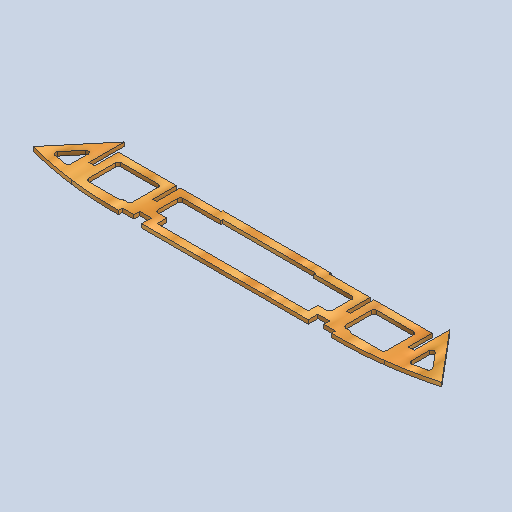
# Autodesk Inventor part: bulkhead_b2
Saved by Autodesk Inventor 2022 (Build 260153070, 153G)
## iProperties
Created: 2021-04-24
Part Number: bulkhead_b2
Material: Plywood, Sheathing, Glazed
Document SubType Name: Modeling
Designer: kardo
Density: 0.75 g/cm^3
Appearance: Plywood - New(2)
Mass: 3.53405 g
Surface Area: 67.3675 cm^2
Volume: 4.71206 cm^3
Author: kardo
Autodesk Inventor part; units mm, degrees
ref_plane "YZ Plane" through (0, 0, 0) normal (1, 0, 0) x (0, 1, 0)
ref_plane "XZ Plane" through (0, 0, 0) normal (0, 1, 0) x (-1, 0, 0)
ref_plane "XY Plane" through (0, 0, 0) normal (0, 0, 1) x (1, 0, 0)
derived "frame_outline.ipt"
sketch "bh_b2" plane through (0, -242, 0) normal (0, 1, 0) x (-1, 0, 0)
  line L0 (0, 19.8309) -> (-30, 19.8309) construction
  line L1 (-30, 19.8309) -> (-30, 20.6564) construction
  line L2 (-30, 20.6564) -> (-81, 20.6564) construction
  line L3 (-81, 20.6564) -> (-81, 10.5173) construction
  line L4 (-81, 10.5173) -> (-106.9114, 41.3973) construction
  line L5 (-105.4998, 40.9597) -> (-81, 11.7619)
  line L6 (0, 20.6309) -> (-28, 20.6309)
  line L7 (-28, 20.6309) -> (-28, 21.4564)
  line L8 (-28, 21.4564) -> (-81, 21.4564)
  line L9 (0, 47.4037) -> (0, 20.6309)
  line L10 (-81, 21.4564) -> (-81, 11.7619)
  spline S0 degree 3 poles (-81, 46.6843) (-83.3296, 46.3773) (-85.8016, 46.0077) (-94.6879, 44.4818) (-100.8447, 43.1089) (-106.9114, 41.3973) knots 2.001746 2.001746 2.001746 2.001746 2.383442 2.383442 3.297577 3.297577 3.297577 3.297577
  spline S1 degree 3 poles (-55, 48.2037) (-56.5728, 48.2037) (-58.0596, 48.1988) (-64.6088, 48.1191) (-71.6624, 47.915) (-81, 46.6843) knots 0 0 0 0 0.47184 0.47184 2.001746 2.001746 2.001746 2.001746
  spline S2 degree 3 poles (0, 48.2037) (-9.1667, 48.2037) (-18.3333, 48.2037) (-36.6667, 48.2037) (-45.8333, 48.2037) (-55, 48.2037) knots 0 0 0 0 2.75 2.75 5.5 5.5 5.5 5.5
  spline S3 degree 3 poles (0, 47.4037) (-1.5278, 47.4037) (-4.5833, 47.4037) (-8.4028, 47.4037) (-12.2222, 47.4037) (-15.2778, 47.4037) (-19.0972, 47.4037) (-22.1528, 47.4037) (-25.9722, 47.4037) (-29.0278, 47.4037) (-32.8472, 47.4037) (-35.9028, 47.4037) (-40.4861, 47.4037) (-46.5972, 47.4037) (-51.9444, 47.4037) (-55, 47.4037) knots 0 0 0 0 0.458333 0.916667 1.145833 1.604167 1.833333 2.291667 2.520833 2.979167 3.208333 3.666667 3.895833 4.583333 5.5 5.5 5.5 5.5
  spline S4 degree 3 poles (-55, 47.4037) (-55.2777, 47.4037) (-55.8277, 47.4034) (-56.5054, 47.402) (-57.1788, 47.3996) (-57.7152, 47.3969) (-58.3187, 47.3928) (-58.722, 47.3894) (-59.1266, 47.3854) (-59.3974, 47.3824) (-59.7371, 47.3783) (-60.0133, 47.3747) (-60.3642, 47.3696) (-60.6495, 47.3651) (-61.0842, 47.3576) (-61.5281, 47.3491) (-62.2112, 47.3344) (-62.8367, 47.3188) (-63.6418, 47.2958) (-64.3045, 47.2744) (-65.3265, 47.2372) (-66.386, 47.1927) (-68.0464, 47.1096) (-69.5986, 47.0164) (-71.6355, 46.871) (-73.3429, 46.7297) (-75.5759, 46.5174) (-77.9084, 46.268) (-79.8817, 46.0248) (-80.8955, 45.8912) knots 0 0 0 0 0.083406 0.166812 0.208515 0.291921 0.333624 0.396179 0.41703 0.458733 0.479585 0.521288 0.542139 0.583842 0.604694 0.667249 0.708952 0.792358 0.834061 0.917467 0.95917 1.084279 1.167685 1.334497 1.417903 1.584715 1.668121 1.834933 2.001746 2.001746 2.001746 2.001746
  spline S5 degree 3 poles (-80.8955, 45.8912) (-81.5213, 45.8087) (-82.7935, 45.6346) (-84.4358, 45.3927) (-85.865, 45.1704) (-86.7205, 45.0322) (-87.4128, 44.9174) (-87.7609, 44.8589) (-88.1986, 44.7845) (-88.5505, 44.7239) (-88.9894, 44.6474) (-89.3405, 44.5854) (-89.8666, 44.4914) (-90.3922, 44.396) (-91.1795, 44.2502) (-91.8784, 44.1178) (-92.9251, 43.9148) (-93.9698, 43.706) (-95.5329, 43.382) (-96.9184, 43.0821) (-98.9907, 42.6143) (-101.7434, 41.9582) (-104.1368, 41.3335) (-105.4998, 40.9597) knots 2.001746 2.001746 2.001746 2.001746 2.104714 2.207682 2.259166 2.323522 2.336393 2.362135 2.375006 2.400748 2.413619 2.439361 2.452232 2.490845 2.516587 2.568071 2.593813 2.67104 2.722524 2.825492 2.876976 3.031429 3.237366 3.237366 3.237366 3.237366
  point P0 (0, 0)
  point P1 (-81, 33.6806)
extrude "Extrusion1" add sketch "bh_b2" along normal blind 2
sketch "Sketch2" plane through (0, -242, 47.4037) normal (0, -1, 0) x (1, 0, 0)
  line L0 (81, -35.6418) -> (81, -25.9472) projected
  line L1 (81, -25.9472) -> (81, -13.7231)
  line L2 (81, -13.7231) -> (84, -13.7231)
  line L3 (84, -13.7231) -> (84, -32.0665)
  line L4 (105.4998, -6.444) -> (81, -35.6418) projected
  point P0 (0, -47.4037)
  dimension "d3" = 3
  constraints: 6 end point, 2 point on line, 1 collinear, 1 horizontal, 1 parallel
  measures "d3" distance between parallel lines of L3 L0
sketch "Sketch3" plane through (0, -242, 47.4037) normal (0, -1, 0) x (1, 0, 0)
  line L0 (0, 0) -> (55, 0) projected
  line L1 (0, 0) -> (55, 0) projected
  line L2 (55, 0) -> (55, -2)
  line L3 (55, -2) -> (49, -2)
  line L4 (49, -2) -> (49, -5)
  line L5 (49, -5) -> (43, -5)
  line L6 (43, -5) -> (43, 0)
  point P0 (0, -47.4037)
  dimension "d4" = 5
  dimension "d5" = 2
  dimension "d6" = 6
  dimension "d7" = 6
  constraints: 10 end point, 3 vertical, 2 horizontal, 1 point on line
  measures "d4" distance of L5.end L6.end
  measures "d5" distance of L0.end L2.end
  measures "d6" distance of L2.end L3.end
  measures "d7" distance of L4.end L5.end
extrude "Extrusion2" cut sketch "Sketch2" against normal through all
extrude "Extrusion3" cut sketch "Sketch3" against normal through all
sketch "Sketch4" plane through (0, -242, 20.6309) normal (0, -1, 0) x (1, 0, 0)
  line L0 (84, 13.0497) -> (84, -5.2937) projected
  line L1 (105.4998, 20.3288) -> (84, -5.2937) projected
  line L2 (88, 20.1303) -> (88, 5.6962)
  line L3 (88, 5.6962) -> (98.344, 18.0237)
  line L4 (98.344, 18.0237) -> (88, 20.1303)
  line L5 (88, 20.1303) -> (88.7982, 24.0498)
  line L6 (98.344, 18.0237) -> (99.1422, 21.9433)
  point P0 (0, -20.6309)
  dimension "d13" = 4
  dimension "d14" = 4
  dimension "d15" = 4
  constraints: 10 end point, 3 parallel, 2 perpendicular, 3 other
  measures "d13" distance of L3.end L6.end
  measures "d14" distance between parallel lines of L1 L3
  measures "d15" distance between parallel lines of L0 L2
sketch "Sketch5" plane through (0, -242, 20.6309) normal (0, -1, 0) x (1, 0, 0)
  line L0 (55, 26.7728) -> (55, 24.7728) projected
  line L1 (81, 0.8256) -> (81, 13.0497) projected
  line L2 (81, 0.8256) -> (28, 0.8256) projected
  line L3 (55, 20.7728) -> (55, 4.8256)
  line L4 (55, 4.8256) -> (77, 4.8256)
  line L5 (77, 4.8256) -> (77, 21.7316)
  line L6 (77, 21.7316) -> (59, 21.7316)
  line L7 (77, 21.7316) -> (77, 25.7316)
  line L8 (49, 24.7728) -> (49, 21.7728) projected
  line L9 (59, 20.7728) -> (55, 20.7728)
  line L10 (59, 21.7316) -> (59, 20.7728)
  line L11 (55, 24.7728) -> (49, 24.7728) projected
  point P0 (0, -20.6309)
  dimension "d16" = 4
  dimension "d17" = 4
  dimension "d19" = 4
  dimension "d34" = 6
  dimension "d35" = 4
  dimension "d36" = 4
  constraints: 14 end point, 5 parallel, 2 collinear, 2 other
  measures "d16" distance of L5.end L7.end
  measures "d17" distance between parallel lines of L1 L5
  measures "d19" distance between parallel lines of L2 L4
  measures "d34" distance between parallel lines of L3 L8
  measures "d35" distance between parallel lines of L11 L9
  measures "d36" distance between parallel lines of L0 L10
sketch "Sketch6" plane through (0, -242, 20.6309) normal (0, -1, 0) x (1, 0, 0)
  line L0 (0, 26.7728) -> (43, 26.7728) projected
  line L1 (55, 26.7728) -> (55, 24.7728) projected
  line L2 (49, 21.7728) -> (43, 21.7728) projected
  line L3 (43, 21.7728) -> (43, 26.7728) projected
  line L4 (81, 0.8256) -> (28, 0.8256) projected
  line L5 (28, 0) -> (0, 0) projected
  line L6 (28, 0.8256) -> (28, 0) projected
  line L7 (0, 0) -> (0, 26.7728) projected
  line L8 (0, 22.7728) -> (39, 22.7728)
  line L9 (39, 22.7728) -> (39, 17.7728)
  line L10 (39, 17.7728) -> (45, 17.7728)
  line L11 (45, 17.7728) -> (45, 4.8256)
  line L12 (45, 4.8256) -> (24, 4.8256)
  line L13 (24, 4.8256) -> (24, 4)
  line L14 (24, 4) -> (0, 4)
  line L15 (49, 24.7728) -> (49, 21.7728) projected
  point P0 (0, -20.6309)
  dimension "d20" = 4
  dimension "d21" = 4
  dimension "d22" = 4
  dimension "d23" = 4
  dimension "d25" = 4
  dimension "d26" = 4
  dimension "d37" = 4
  constraints: 14 end point, 7 parallel, 2 point on line
  measures "d20" distance between parallel lines of L0 L8
  measures "d21" distance between parallel lines of L5 L14
  measures "d22" distance between parallel lines of L6 L13
  measures "d23" distance between parallel lines of L4 L12
  measures "d25" distance between parallel lines of L10 L2
  measures "d26" distance between parallel lines of L3 L9
  measures "d37" distance between parallel lines of L11 L15
extrude "Extrusion4" cut sketch "Sketch4" against normal through all
extrude "Extrusion5" cut sketch "Sketch6" against normal through all
extrude "Extrusion6" cut sketch "Sketch5" against normal through all
fillet "Fillet1" radius 1.3333 11 edges at (55, -241, 25.4564) (88, -241, 26.3271) (98.344, -241, 38.6546) (77, -241, 42.3625) (77, -241, 25.4564) (55, -241, 41.4037) (88, -241, 40.7611) (45, -241, 25.4564) (45, -241, 38.4037) (59, -241, 41.4037) (59, -241, 42.3625)
sketch "Sketch7" plane through (0, -242, 20.6309) normal (0, -1, 0) x (1, 0, 0)
  line L0 (49, 0.8093) -> (49, 13.0497)
  line L1 (49, 13.0497) -> (51, 13.0497)
  line L2 (51, 13.0497) -> (51, 0.8256)
  line L3 (81, 0.8256) -> (28, 0.8256) projected
  line L4 (81, 13.0497) -> (84, 13.0497) projected
  line L5 (49, 24.7728) -> (49, 21.7728) projected
  point P0 (0, -20.6309)
  point P1 (49, 0.8256)
  dimension "d38" = 2
  constraints: 6 end point, 2 collinear, 2 vertical, 1 horizontal, 1 point on line
  measures "d38" distance between parallel lines of L0 L2
extrude "Extrusion7" cut sketch "Sketch7" against normal through all
mirror "Mirror1" about plane through (0, 0, 0) normal (1, 0, 0)
equation "\"d1\" = bulkhead_thickness"
equation "\"d3\" = stringer_thickness"
equation "\"d4\" = cowl_insulation_thickness + cowl_liner_thickness"
equation "\"d5\" = cowl_liner_thickness"
equation "\"d6\" = cowl_liner_width"
equation "\"d7\" = cowl_insulation_width"
equation "\"d13\" = inset"
equation "\"d14\" = inset"
equation "\"d15\" = inset"
equation "\"d16\" = inset"
equation "\"d17\" = inset"
equation "\"d19\" = inset"
equation "\"d34\" = inset + bulkhead_thickness"
equation "\"d35\" = inset"
equation "\"d36\" = inset"
equation "\"d20\" = inset"
equation "\"d21\" = inset"
equation "\"d22\" = inset"
equation "\"d23\" = inset"
equation "\"d25\" = inset"
equation "\"d26\" = inset"
equation "\"d37\" = inset"
equation "\"d33\" = 0.333333 * inset"
equation "\"d38\" = bulkhead_thickness"
equation "\"bulkhead_thickness\" = 2"
equation "\"stringer_thickness\" = 3"
equation "\"cowl_insulation_thickness\" = 3"
equation "\"cowl_liner_thickness\" = 2"
equation "\"cowl_liner_width\" = 6"
equation "\"cowl_insulation_width\" = 6"
equation "\"inset\" = 4"
body "Solid1"
